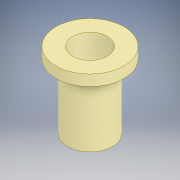
# Autodesk Inventor part: HSHW-M5-6.6-N
Saved by Autodesk Inventor 2019 (Build 230136000, 136)
## iProperties
Created: 2018-05-06
Part Number: HSHW-M5-6.6-N
Material: Nylon 6/6
Document SubType Name: Modeling
Designer: IEUser
Density: 1.13 g/cm^3
Appearance: Nylon 6
Author: IEUser
Autodesk Inventor part; units mm, degrees
ref_plane "YZ Plane" through (0, 0, 0) normal (1, 0, 0) x (0, 1, 0)
ref_plane "XZ Plane" through (0, 0, 0) normal (0, 1, 0) x (-1, 0, 0)
ref_plane "XY Plane" through (0, 0, 0) normal (0, 0, 1) x (1, 0, 0)
sketch "Washer Cross Section" plane through (0, 0, 0) normal (0, 1, 0) x (-1, 0, 0)
  circle A0 centre (0, 0) radius 3.3
  dimension "d0" = 6.6
  constraints: 1 centre point, 1 coincident
  measures "d0" diameter of A0
extrude "Washer" add sketch "Washer Cross Section" against normal blind 9.53
sketch "Shoulder Cross Section" plane through (0, 0, 0) normal (0, 1, 0) x (1, 0, 0)
  circle A0 centre (0, 0) radius 5
  dimension "d3" = 10
  constraints: 1 centre point, 1 coincident
  measures "d3" diameter of A0
extrude "Shoulder" add sketch "Shoulder Cross Section" along normal blind 1.6
sketch "Screw Hole Position" plane through (0, 1.6, 0) normal (0, 1, 0) x (1, 0, 0)
  point P0 (0, 0)
  point P1 (0, 0)
  constraints: 1 coincident
hole "Screw Hole" at (0, 1.6, 0) direction (0, -1, 0) diameter 5.08 end through all
body "Solid1"
